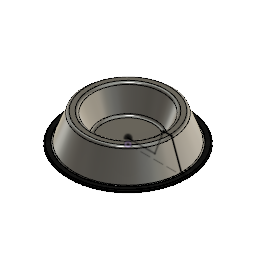
Day #11 Dog Bowl v3 (Autodesk Fusion 360 design; units mm, degrees)
Autodesk Fusion 360 part; units mm, degrees
sketch "Bowl Sketch" plane through (0, 0, 0) normal (0, 1, 0) x (1, 0, 0)
  line L0 (0, 0) -> (110, 0) construction
  line L1 (110, 0) -> (110, -2.5)
  line L2 (110, -2.5) -> (100, -2.5)
  line L3 (100, -2.5) -> (81.1889, -54.1831)
  line L4 (81.1889, -54.1831) -> (66.1889, -54.1831)
  line L5 (66.1889, -54.1831) -> (50.1076, -10)
  line L6 (0, -10) -> (50.1076, -10)
  dimension "d1" = 110
  dimension "d2" = 10
  dimension "d3" = 110
  dimension "d4" = 55
  dimension "d5" = 2.5
  dimension "d6" = 15
  dimension "d7" = 10
  dimension "d8" = 110
  constraint coincident L0.start origin
  constraint horizontal L0
  constraint perpendicular L0 L1
  constraint perpendicular L1 L2
  constraint parallel L2 L4
  constraint parallel L0 L6
  constraint vertical L0.start L6.start
  measures "d1" distance of L0.start L0.end
  measures "d2" distance of L1.end L2.end
  measures "d3" angle of L2 L3
  measures "d4" distance of L2.end L3.end
  measures "d5" distance of L0 L2
  measures "d6" distance of L3.end L4.end
  measures "d7" distance of L0 L6
  measures "d8" angle of L5 L6
surface "Revolve1" add revolved angle 360 about axis through (0, 0, 1.75) along (0, 0, 20.75) path "Bowl Sketch" along L1 L2 L3 L4 L5 L6 makes body 1
fillet "Fillet1" radius 5 3 edges at (-61.7097, -23.9349, 54.1831) (-75.6946, -29.3592, 54.1831) (-46.7166, -18.1197, 10) on bodies 1
fillet "Fillet1" radius 2.5 1 edges at (-93.2327, -36.1615, 2.5) on bodies 1
thicken "Thicken1" add thickness -2.5 9 faces at (-34.2433, -87.2505, 19.7277) (68.6023, -41.922, 53.3853) (74.4732, -7.3218, 54.1831) (67.3158, -17.1407, 54.178) (13.7852, -60.3968, 42.5369) (50.2072, -10.1496, 13.0791) (8.8256, 11.0669, 10) (-76.3154, 64.0363, 3.6876) (106.8406, -5.4649, 2.5) separate body on bodies 1 makes body 2
fillet "Fillet2" radius 0.5 2 edges at (-102.556, -39.7777, 2.5) (-102.556, -39.7777, 0) on bodies 2
offset_surface "SurfaceOffset1" offset 0.5 5 faces at (-13.6695, -109.0798, 2.25) (106.1303, -10.4951, 2.5) (19.1013, -108.3289, 1) (87.6312, 66.378, 0.25) (106.1303, -10.4951, 0) on bodies 2 makes body 3
thicken "Thicken2" add thickness 1 surfaces 3 separate body makes body 4
hidden bodies 3
named bodies: "Bowl Surface Body", "Bowl Solid Body"
